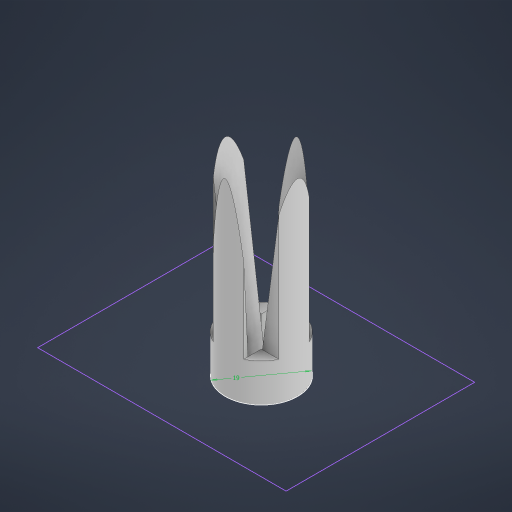
# Autodesk Inventor part: muzzle light
Saved by Autodesk Inventor 2024.3 (Build 283343000, 343)
## iProperties
Created: 2025-08-05
Part Number: muzzle light
Material: Generic
Document SubType Name: Modeling
Designer: giuseppe
Density: 1 g/cm^3
Appearance: Default
Author: giuseppe
## iProperties of the stored document muzzle light_3DPrint.ipt
Created: 2025-08-06
Part Number: muzzle light_3DPrint
Material: Generic
Document SubType Name: Modeling
Designer: giuseppe
Density: 1 g/cm^3
Appearance: Default
Author: giuseppe
Autodesk Inventor part; units mm, degrees
ref_plane "YZ Plane" through (0, 0, 0) normal (1, 0, 0) x (0, 1, 0)
ref_plane "XZ Plane" through (0, 0, 0) normal (0, 1, 0) x (-1, 0, 0)
ref_plane "XY Plane" through (0, 0, 0) normal (0, 0, 1) x (1, 0, 0)
sketch "Sketch1" plane through (0, 0, 0) normal (0, 1, 0) x (-1, 0, 0)
  circle A0 centre (0, 0) radius 9.5
  line L0 (35.7937, -26.5264) -> (-29.5588, -26.5264)
  line L1 (-29.5588, -26.5264) -> (-29.5588, 23.0689)
  line L2 (-29.5588, 23.0689) -> (35.7937, 23.0689)
  line L3 (35.7937, 23.0689) -> (35.7937, -26.5264)
  dimension "d0" = 19
  constraints: 8 end point, 2 parallel, 1 centre point, 1 coincident, 1 horizontal, 1 perpendicular
  measures "d0" diameter of A0
sketch "Sketch2" plane through (0, 0, 0) normal (0, 0, 1) x (1, 0, 0)
  line L0 (9.5, 0) -> (9.5, 53.7589) construction
  line L1 (0, 0) -> (3, 0) construction
  line L2 (3, 0) -> (9.5, 49.5757)
  line L3 (9.5, 0) -> (-9.5, 0) construction
  line L4 (3, 0) -> (9.5, 0)
  line L5 (9.5, 0) -> (9.5, 49.5757)
  dimension "d2" = 3
  dimension "d3" = 50
  constraints: 10 end point, 2 collinear, 1 horizontal, 1 point on line, 1 vertical
  measures "d2" distance of L1.start L1.end
  measures "d3" distance of L1.end L2.end
extrude "Extrusion1" add sketch "Sketch2" along normal mid plane 8
mirror "Mirror1" about plane through (0, 0, 0) normal (1, 0, 0) of "Extrusion1"
sketch "Sketch3" plane through (0, 0, 0) normal (1, 0, 0) x (0, 1, 0)
  line L0 (0, -9.5) -> (0, 9.5) projected
  line L1 (0, 9.5) -> (49.5757, 9.5)
  line L2 (0, 4) -> (49.5757, 4) projected
  line L3 (49.5757, 4) -> (49.5757, -4) projected
  line L4 (0, 4) -> (49.5757, 4) projected
  line L5 (0, -4) -> (0, 4) projected
  line L6 (49.5757, -4) -> (0, -4) projected
  line L7 (0, 4) -> (49.5757, 4) projected
  line L8 (49.5757, 9.5) -> (0, 7)
  line L9 (0, 9.5) -> (0, 4)
  point P0 (0, 0)
  dimension "d15" = 3
  constraints: 6 end point, 2 parallel, 1 collinear, 1 point on line
  measures "d15" distance of L2.start L8.end
extrude "Extrusion2" add sketch "Sketch3" along normal mid plane 8 contours L0 L1 L8
mirror "Mirror2" about plane through (0, 0, 0) normal (0, 0, 1) of "Extrusion2"
sketch "Sketch7" plane through (3, 0, 4) normal (0, -1, 0) x (1, 0, 0)
  circle A0 centre (-3, -4) radius 9.5 projected
  line L0 (0, -8) -> (0, 0) projected
  line L1 (0, -8) -> (0, -11)
  line L2 (1, -13.5) -> (1, -11) projected
  line L3 (0, -11) -> (1, -11)
  line L4 (-7, -11) -> (1, -11) projected
  line L5 (-7, -11) -> (-6, -11)
  line L6 (-6, -8) -> (-6, 0) projected
  line L7 (-6, -11) -> (-6, -8)
  line L8 (-7, 3) -> (1, 3) projected
  line L9 (-7, 3) -> (-6, 3)
  line L10 (-6, 3) -> (-6, 0)
  line L11 (1, 3) -> (0, 3)
  line L12 (6.5, 0) -> (0, 0) projected
  line L13 (0, 3) -> (0, 0)
  line L14 (12.4541, -14.5863) -> (-21.2627, -14.5863)
  line L15 (-21.2627, -14.5863) -> (-21.2627, 9.286)
  line L16 (-21.2627, 9.286) -> (12.4541, 9.286)
  line L17 (12.4541, 9.286) -> (12.4541, -14.5863)
  line L18 (6.5, -8) -> (6.5, 0) projected
  line L19 (0, 0) -> (6.5, 0) projected
  line L20 (0, -8) -> (0, 0) projected
  line L21 (6.5, -8) -> (0, -8) projected
  line L22 (-7, -11) -> (1, -11) projected
  line L23 (-7, -11) -> (-7, -13.5) projected
  line L24 (1, -13.5) -> (-7, -13.5) projected
  line L25 (1, -13.5) -> (1, -11) projected
  line L26 (-12.5, -8) -> (-12.5, 0) projected
  line L27 (-12.5, -8) -> (-6, -8) projected
  line L28 (-6, -8) -> (-6, 0) projected
  line L29 (-6, 0) -> (-12.5, 0) projected
  line L30 (1, 3) -> (1, 0)
  line L31 (1, -11) -> (1, -8)
  line L32 (-7, -11) -> (-7, -8)
  line L33 (-7, 3) -> (-7, 0)
  line L34 (-7, 3) -> (1, 3) projected
  line L35 (1, 5.5) -> (1, 3) projected
  line L36 (1, 5.5) -> (-7, 5.5) projected
  line L37 (-7, 3) -> (-7, 5.5) projected
  point P0 (-7, 4.6168)
  point P1 (-11.6168, 0)
  point P2 (-11.6168, -8)
  point P3 (-7, -12.6168)
  point P4 (1, -12.6168)
  point P5 (5.6168, -8)
  point P6 (1, 4.6168)
  point P7 (5.6168, 0)
  point P8 (-12.5, -4)
  point P9 (-3, -13.5)
  point P10 (6.5, -4)
  point P11 (-3, 5.5)
  constraints: 32 end point, 6 point on line, 5 perpendicular, 4 collinear, 2 horizontal, 2 parallel, 1 vertical
extrude "Extrusion6" add sketch "Sketch7" against normal blind 10 contours L12 L30 L35 A0 | A0 L2 L31 L21 | L37 L33 L29 A0 | A0 L27 L32 L23
extrude "Extrusion7" cut sketch "Sketch7" against normal through all contours L18 L21 A0 | A0 L12 L18 | A0 L36 L35 | L2 L24 A0 | A0 L37 L36 | L24 L23 A0 | A0 L26 L29 | L27 L26 A0
sketch "Sketch4" plane through (0, 0, 0) normal (0, 1, 0) x (-1, 0, 0)
  line L0 (3, -2.5) -> (3, 2.5) projected
  line L1 (3, -2.5) -> (9.5, -2.5) projected
  line L2 (9.5, 2.5) -> (9.5, -2.5) projected
  line L3 (9.5, 2.5) -> (3, 2.5) projected
  line L4 (2.5, -9.5) -> (-2.5, -9.5) projected
  line L5 (2.5, -9.5) -> (2.5, -2.5) projected
  line L6 (2.5, -2.5) -> (-2.5, -2.5) projected
  line L7 (-2.5, -2.5) -> (-2.5, -9.5) projected
  line L8 (-3, -2.5) -> (-3, 2.5) projected
  line L9 (-9.5, 2.5) -> (-3, 2.5) projected
  line L10 (-9.5, 2.5) -> (-9.5, -2.5) projected
  line L11 (-3, -2.5) -> (-9.5, -2.5) projected
  line L12 (2.5, 9.5) -> (-2.5, 9.5) projected
  line L13 (-2.5, 2.5) -> (-2.5, 9.5) projected
  line L14 (2.5, 2.5) -> (-2.5, 2.5) projected
  line L15 (2.5, 9.5) -> (2.5, 2.5) projected
  circle A0 centre (0, 0) radius 9.5 projected
  point P0 (-2.5, 9.1652)
  point P1 (-9.1652, 2.5)
  point P2 (9.1652, 2.5)
  point P3 (2.5, 9.1652)
  point P4 (-9.1652, -2.5)
  point P5 (-2.5, -9.1652)
  point P6 (2.5, -9.1652)
  point P7 (9.1652, -2.5)
  point P8 (-9.5, 0)
  point P9 (0, 9.5)
  point P10 (9.5, 0)
  point P11 (0, -9.5)
sketch "Sketch5" plane through (0, 46.25, 0) normal (0, 1, 0) x (1, 0, 0)
  line L0 (-22.7288, -35.2268) -> (16.9474, -35.2268)
  line L1 (16.9474, -35.2268) -> (16.9474, 22.5304)
  line L2 (16.9474, 22.5304) -> (-22.7288, 22.5304)
  line L3 (-22.7288, 22.5304) -> (-22.7288, -35.2268)
  point P0 (0, 0)
  constraints: 8 end point, 2 parallel, 1 horizontal, 1 perpendicular
body "Solid1"
